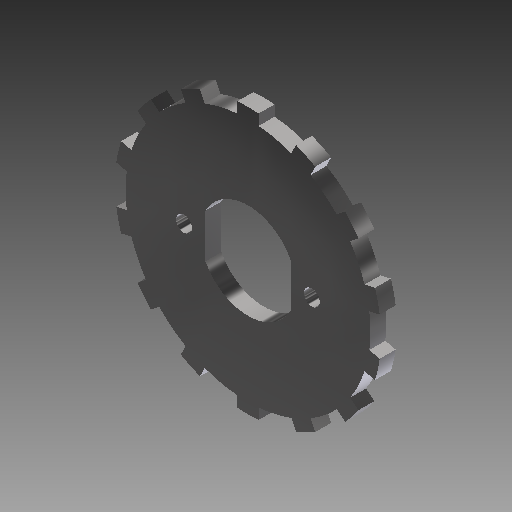
# Autodesk Inventor part: 404-03
Saved by Autodesk Inventor 2019 (Build 230136000, 136)
## iProperties
Company: Autodesk Inc.
Created: 2017-06-27
Part Number: 404-03
Material: Steel, Mild
Document SubType Name: Modeling
Designer: Autodesk Inc.
Mass: 4.46434 g
Surface Area: 9.64868 cm^2
Volume: 0.568706 cm^3
Density: 7.85 g/cm^3
Appearance: Semi-Polished
Author: Inventor
Autodesk Inventor part; units mm, degrees
ref_plane "YZ Plane" through (0, 0, 0) normal (1, 0, 0) x (0, 1, 0)
ref_plane "XZ Plane" through (0, 0, 0) normal (0, 1, 0) x (-1, 0, 0)
ref_plane "XY Plane" through (0, 0, 0) normal (0, 0, 1) x (1, 0, 0)
sketch "Sketch1" plane through (0, 0, 0) normal (0, 0, 1) x (1, 0, 0)
  line L0 (0, 0) -> (-2.559, 11.2117)
  line L1 (0, 0) -> (2.559, 11.2117)
  line L2 (0, 0) -> (0, 11.5) construction
  line L3 (-1, 11.4564) -> (-1, 12.4599)
  line L4 (1, 11.4564) -> (1, 12.4599)
  line L5 (-1, 12.4599) -> (1, 12.4599) construction
  arc A0 (1, 12.4599) -> (-1, 12.4599) centre (0, 0) ccw
  line L6 (-1, 11.4564) -> (1, 11.4564) construction
  arc A1 (2.559, 11.2117) -> (1, 11.4564) centre (0, 0) ccw
  arc A2 (-1, 11.4564) -> (-2.559, 11.2117) centre (0, 0) ccw
  line L7 (-2.559, 11.2117) -> (2.559, 11.2117) construction
  point P0 (0, 12.5)
  point P1 (0, 12.4599)
  dimension "d0" = 25.714
  dimension "d2" = 12.5
  dimension "d3" = 2
  dimension "d4" = 11.5
  constraints: 17 end point, 7 point on circle, 3 centre point, 2 parallel, 2 perpendicular, 2 vertical alignment, 1 coincident, 1 horizontal, 1 midpoint, 1 vertical
  measures "d0" angle of L1 L0
  measures "d2" radius of A0
  measures "d3" distance between parallel lines of L3 L4
  measures "d4" radius of A1
extrude "Extrusion1" add sketch "Sketch1" along normal mid plane 1.5
pattern_circular "Circular Pattern1" count 14 over 360 about axis through (0, 0, -0.75) along (0, 0, 1)
sketch "Sketch2" plane through (0, 0, 0.75) normal (0, 0, 1) x (1, 0, 0)
  circle A0 centre (0, 0) radius 4.5
  line L0 (-4, 2.0616) -> (-4, -2.0616)
  line L1 (4, 2.0616) -> (4, -2.0616)
  dimension "d10" = 9
  dimension "d11" = 8
  constraints: 4 end point, 4 point on circle, 2 parallel, 1 centre point, 1 coincident, 1 vertical
  measures "d10" diameter of A0
  measures "d11" distance between parallel lines of L1 L0
extrude "Extrusion2" cut sketch "Sketch2" against normal through all contours L1 A0 L0
sketch "Sketch3" plane through (0, 0, 0.75) normal (0, 0, 1) x (1, 0, 0)
  line L0 (-6, 0) -> (6, 0) construction
  point P0 (0, 0)
  point P1 (0, 0)
  dimension "d14" = 12
  constraints: 2 end point, 1 coincident, 1 horizontal, 1 midpoint
  measures "d14" distance of L0.start L0.end
hole "Hole1" at (-6, 0, 0.75) at (6, 0, 0.75) direction (0, 0, -1) diameter 1.5 end through all
body "Solid1"
